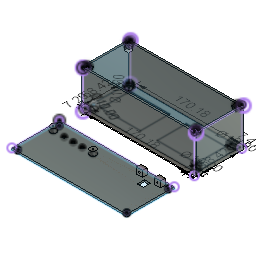
Digital Clock Enclosure v22 (Autodesk Fusion 360 design; units mm, degrees)
Autodesk Fusion 360 part; units mm, degrees
note: some values were not read from the file. Chosen so that the rebuilt part matches the saved one: which face or edge a step refers to.
sketch "Sketch1" plane through (0, 0, 0) normal (0, 0, 1) x (1, 0, 0)
  line L0 (0, 0) -> (185, 0)
  line L1 (185, 0) -> (185, 73)
  line L2 (185, 73) -> (0, 73)
  line L3 (0, 73) -> (0, 0)
  line L4 (13, 62) -> (78.5, 62)
  line L5 (78.5, 62) -> (78.5, 14)
  line L6 (78.5, 14) -> (13, 14)
  line L7 (13, 14) -> (13, 62)
  line L8 (106.5, 62) -> (172, 62)
  line L9 (172, 62) -> (172, 14)
  line L10 (172, 14) -> (106.5, 14)
  line L11 (106.5, 14) -> (106.5, 62)
  dimension "d1" = 185
  dimension "d2" = 73
  dimension "d3" = 13
  dimension "d4" = 13
  dimension "d5" = 28
  dimension "d6" = 14
  dimension "d7" = 14
  dimension "d8" = 11
  dimension "d9" = 11
  constraint horizontal L0
  constraint vertical L1
  constraint horizontal L2
  constraint vertical L3
  constraint coincident L0.start L3.end
  constraint horizontal L4
  constraint vertical L5
  constraint horizontal L6
  constraint vertical L7
  constraint horizontal L8
  constraint vertical L9
  constraint horizontal L10
  constraint vertical L11
  constraint equal L6 L10
  measures "d1" distance of L1 L3
  measures "d2" distance of L0.end L1.end
  measures "d3" distance of L1 L9
  measures "d4" distance of L3 L7
  measures "d5" distance of L5 L11
  measures "d6" distance of L0 L10
  measures "d7" distance of L0 L6
  measures "d8" distance of L2 L8
  measures "d9" distance of L2 L4
extrude "Extrude1" add sketch "Sketch1" along normal blind 60 makes body 1
shell "Shell2" thickness 3 outward yes removed faces 1 at (97.1667, 30, 60) on bodies 1
extrude "Extrude6" cut 1 faces at (129.3333, 61, 60) along direction (0, 0, -1) blind 63 on bodies 1 bodies 1
extrude "Extrude7" cut 1 faces at (55.6667, 15, 60) along direction (0, 0, -1) blind 63 on bodies 1 bodies 1
sketch "Sketch5" plane through (0, 0, 0) normal (0, 0, 1) x (-1, 0, 0)
  line L0 (-78.5, -14) -> (-13, -14)
  line L1 (-13, -14) -> (-13, -62)
  line L2 (-13, -62) -> (-78.5, -62)
  line L3 (-78.5, -62) -> (-78.5, -14)
  line L4 (-172, -14) -> (-106.5, -14)
  line L5 (-106.5, -14) -> (-106.5, -62)
  line L6 (-106.5, -62) -> (-172, -62)
  line L7 (-172, -62) -> (-172, -14)
  line L8 (0, -73) -> (0, 0)
  line L9 (0, 0) -> (-185, 0)
  line L10 (-185, 0) -> (-185, -73)
  line L11 (-185, -73) -> (0, -73)
  circle A0 centre (-7.41, -65.71) radius 5
  circle A1 centre (-7.41, -7.29) radius 5
  circle A2 centre (-177.59, -65.71) radius 5
  circle A3 centre (-177.59, -7.29) radius 5
  dimension "d26" = 10
  dimension "d27" = 10
  dimension "d28" = 10
  dimension "d29" = 10
  dimension "d30" = 170.18
  dimension "d31" = 170.18
  dimension "d32" = 58.42
  dimension "d33" = 58.42
  dimension "d34" = 7.41
  dimension "d35" = 7.41
  dimension "d36" = 7.29
  dimension "d37" = 7.29
  measures "d26" diameter of A0
  measures "d27" diameter of A1
  measures "d28" diameter of A2
  measures "d29" diameter of A3
  measures "d30" horizontal distance of A0.centre A2.centre
  measures "d31" horizontal distance of A1.centre A3.centre
  measures "d32" vertical distance of A2.centre A3.centre
  measures "d33" vertical distance of A0.centre A1.centre
  measures "d34" distance of L10 A2.centre
  measures "d35" distance of L10 A3.centre
  measures "d36" distance of L9 A3.centre
  measures "d37" distance of L9 A1.centre
extrude "Extrude8" add sketch "Sketch5" along normal blind 5 contours A0 | A1 | A2 | A3 bodies 1
sketch "Sketch10" plane through (0, 0, 0) normal (0, 0, 1) x (-1, 0, 0)
  circle A0 centre (-7.41, -65.71) radius 5
  circle A1 centre (-7.41, -7.29) radius 5
  circle A2 centre (-177.59, -65.71) radius 5
  circle A3 centre (-177.59, -7.29) radius 5
  line L0 (-78.5, -14) -> (-13, -14)
  line L1 (-13, -14) -> (-13, -62)
  line L2 (-13, -62) -> (-78.5, -62)
  line L3 (-78.5, -62) -> (-78.5, -14)
  line L4 (-172, -14) -> (-106.5, -14)
  line L5 (-106.5, -14) -> (-106.5, -62)
  line L6 (-106.5, -62) -> (-172, -62)
  line L7 (-172, -62) -> (-172, -14)
  line L8 (0, -73) -> (0, 0)
  line L9 (0, 0) -> (-185, 0)
  line L10 (-185, 0) -> (-185, -73)
  line L11 (-185, -73) -> (0, -73)
extrude "Extrude9" cut 1 faces at (5.9084, 66.4331, 5) along direction (0, 0, -1) blind 5 on bodies 1 bodies 1
sketch "Sketch11" plane through (0, 0, 0) normal (0, 0, 1) x (-1, 0, 0)
extrude "Extrude10" cut 3 faces at (176.2129, 65.2679, 5) (178.4699, 5.0481, 5) (8.3568, 6.5995, 5) along direction (0, 0, -1) blind 5 on bodies 1 bodies 1
sketch "Sketch12" plane through (0, 0, 0) normal (0, 0, 1) x (1, 0, 0)
extrude "Extrude11" add sketch "Sketch10" along normal blind 5 contours A0 | A1 | A2 | A3 bodies 1
sketch "Sketch13" plane through (0, 0, 0) normal (0, 0, 1) x (-1, 0, 0)
sketch "Sketch14" plane through (0, 0, 0) normal (0, 0, 1) x (-1, 0, 0)
sketch "Sketch15" plane through (0, 0, 0) normal (0, 0, 1) x (-1, 0, 0)
sketch "Sketch16" plane through (0, 0, 0) normal (1, 0, 0) x (0, 1, 0)
  line L0 (0, 0) -> (73, 0)
  line L1 (73, 0) -> (73, 60)
  line L2 (73, 60) -> (0, 60)
  line L3 (0, 60) -> (0, 0)
sketch "Sketch18" plane through (-3, 0, 0) normal (-1, 0, 0) x (0, -1, 0)
  line L0 (-76, -3) -> (3, -3)
  line L1 (3, -3) -> (3, 60)
  line L2 (3, 60) -> (-76, 60)
  line L3 (-76, 60) -> (-76, -3)
sketch "Sketch19" plane through (-3, 0, 0) normal (-1, 0, 0) x (0, -1, 0)
  line L0 (-76, -3) -> (3, -3)
  line L1 (3, -3) -> (3, 60)
  line L2 (3, 60) -> (-76, 60)
  line L3 (-76, 60) -> (-76, -3)
sketch "Sketch20" plane through (0, 0, 0) normal (1, 0, 0) x (0, 1, 0)
  line L0 (0, 0) -> (73, 0)
  line L1 (73, 0) -> (73, 60)
  line L2 (73, 60) -> (0, 60)
  line L3 (0, 60) -> (0, 0)
sketch "Sketch24" plane through (188, 0, 0) normal (1, 0, 0) x (0, 1, 0)
  line L0 (-3, -3) -> (76, -3)
  line L1 (76, -3) -> (76, 60)
  line L2 (76, 60) -> (-3, 60)
  line L3 (-3, 60) -> (-3, -3)
sketch "Sketch25" plane through (188, 0, 0) normal (1, 0, 0) x (0, 1, 0)
sketch "Sketch34" plane through (0, 0, 0) normal (1, 0, 0) x (0, 1, 0)
  line L0 (0, 60) -> (7, 60)
  line L1 (7, 60) -> (7, 55)
  line L2 (7, 55) -> (0, 55)
  line L3 (0, 55) -> (0, 60)
  line L4 (-3, 60) -> (-3, -3)
  point P0 (-3, 60)
  dimension "d68" = 7
  dimension "d69" = 5
  dimension "d70" = 3
  constraint horizontal L0
  constraint vertical L1
  constraint horizontal L2
  constraint vertical L3
  constraint coincident L0 P0
  measures "d68" distance of L0.start L0.end
  measures "d69" distance of L0.start L2.end
  measures "d70" distance of L3 L4
extrude "Extrude15" add sketch "Sketch34" along normal blind 7 bodies 1
move_face "MoveFace7" to x (0.642788, 0, 0.766044) y (-0.439385, 0.819152, 0.368688) z (-0.627507, -0.573576, 0.526541) at (40.0891, 32.8126, 18.0971) 1 faces at (2.3333, 4.6667, 55) on bodies 1
move_face "MoveFace8" by (-1.255, -1.1472, 1.0531) 1 faces at (2.3333, 2.3333, 44.3549) on bodies 1
sketch "Sketch35" plane through (0, 0, 0) normal (1, 0, 0) x (0, 1, 0)
  line L0 (66, 60) -> (73, 60)
  line L1 (73, 60) -> (73, 55)
  line L2 (73, 55) -> (66, 55)
  line L3 (66, 55) -> (66, 60)
  line L4 (76, -3) -> (76, 60)
  point P0 (76, 60)
  dimension "d73" = 7
  dimension "d74" = 5
  dimension "d75" = 3
  constraint horizontal L0
  constraint vertical L1
  constraint horizontal L2
  constraint vertical L3
  constraint coincident L0 P0
  measures "d73" distance of L0.start L0.end
  measures "d74" distance of L0.start L2.end
  measures "d75" distance of L1 L4
extrude "Extrude16" add sketch "Sketch35" along normal blind 7 bodies 1
move_face "MoveFace9" to x (0.642788, 0, 0.766044) y (0.439385, 0.819152, -0.368688) z (-0.627507, 0.573576, 0.526541) at (6.7589, -18.4636, 46.0644) 1 faces at (2.3333, 70.6667, 55) on bodies 1
sketch "Sketch36" plane through (185, 0, 0) normal (-1, 0, 0) x (0, -1, 0)
  line L0 (-73, 0) -> (0, 0)
  line L1 (0, 0) -> (0, 60)
  line L2 (0, 60) -> (-73, 60)
  line L3 (-73, 60) -> (-73, 0)
sketch "Sketch37" plane through (185, 0, 0) normal (-1, 0, 0) x (0, -1, 0)
  line L0 (-73, 60) -> (-66, 60)
  line L1 (-66, 60) -> (-66, 55)
  line L2 (-66, 55) -> (-73, 55)
  line L3 (-73, 55) -> (-73, 60)
  line L4 (-76, 60) -> (-76, -3)
  line L5 (-7, 60) -> (0, 60)
  line L6 (0, 60) -> (0, 55)
  line L7 (0, 55) -> (-7, 55)
  line L8 (-7, 55) -> (-7, 60)
  line L9 (3, -3) -> (3, 60)
  point P0 (-76, 60)
  point P1 (3, 60)
  dimension "d78" = 7
  dimension "d79" = 5
  dimension "d80" = 3
  dimension "d81" = 7
  dimension "d82" = 5
  dimension "d83" = 3
  constraint horizontal L0
  constraint vertical L1
  constraint horizontal L2
  constraint vertical L3
  constraint coincident L0 P0
  constraint horizontal L5
  constraint vertical L6
  constraint horizontal L7
  constraint vertical L8
  constraint coincident L5 P1
  measures "d78" distance of L0.start L0.end
  measures "d79" distance of L0.start L2.end
  measures "d80" distance of L3 L4
  measures "d81" distance of L5.start L5.end
  measures "d82" distance of L5.start L7.end
  measures "d83" distance of L6 L9
extrude "Extrude17" add sketch "Sketch37" along normal blind 7 bodies 1
move_face "MoveFace10" to x (0.642788, 0, -0.766044) y (0.439385, 0.819152, 0.368688) z (0.627507, -0.573576, 0.526541) at (27.2502, 31.6655, 160.8684) 1 faces at (182.6667, 2.3333, 55) on bodies 1
move_face "MoveFace11" to x (0.819152, -0.439385, -0.368688) y (0, 0.642788, -0.766044) z (0.573576, 0.627507, 0.526541) at (1.7914, 68.5287, 143.2787) 1 faces at (182.6667, 68.3333, 55) on bodies 1
sketch "Sketch39" plane through (0, 0, 0) normal (0, 0, 1) x (1, 0, 0)
  line L0 (-0.7205, -41.6473) -> (190.2795, -41.6473)
  line L1 (190.2795, -41.6473) -> (190.2795, -120.6473)
  line L2 (190.2795, -120.6473) -> (-0.7205, -120.6473)
  line L3 (-0.7205, -120.6473) -> (-0.7205, -41.6473)
  dimension "d86" = 191
  dimension "d87" = 79
  constraint horizontal L0
  constraint vertical L1
  constraint horizontal L2
  constraint vertical L3
  measures "d86" distance of L0.start L0.end
  measures "d87" distance of L0.start L2.end
extrude "Extrude18" add sketch "Sketch39" along normal blind 3 separate body makes body 2
sketch "Sketch41" plane through (0, 0, 0) normal (0, 0, -1) x (1, 0, 0)
  line L0 (190.2795, 120.6473) -> (-0.7205, 120.6473)
  line L1 (-0.7205, 120.6473) -> (-0.7205, 41.6473)
  line L2 (-0.7205, 41.6473) -> (190.2795, 41.6473)
  line L3 (190.2795, 41.6473) -> (190.2795, 120.6473)
  circle A0 centre (4.2795, 115.6473) radius 1.6
  circle A1 centre (4.2795, 46.6473) radius 1.6
  circle A2 centre (185.2795, 115.6473) radius 1.6
  circle A3 centre (185.2795, 46.6473) radius 1.6
  dimension "d92" = 3.2
  dimension "d93" = 3.2
  dimension "d94" = 3.2
  dimension "d95" = 3.2
  dimension "d96" = 5
  dimension "d97" = 5
  dimension "d98" = 5
  dimension "d99" = 5
  dimension "d100" = 5
  dimension "d101" = 5
  dimension "d102" = 5
  dimension "d103" = 5
  measures "d92" diameter of A0
  measures "d93" diameter of A1
  measures "d94" diameter of A2
  measures "d95" diameter of A3
  measures "d96" distance of L1 A0.centre
  measures "d97" distance of L0 A0.centre
  measures "d98" distance of L1 A1.centre
  measures "d99" distance of L2 A1.centre
  measures "d100" distance of L3 A3.centre
  measures "d101" distance of L2 A3.centre
  measures "d102" distance of L0 A2.centre
  measures "d103" distance of L3 A2.centre
extrude "Extrude19" cut sketch "Sketch41" against normal blind 3 contours A0 bodies 2
extrude "Extrude20" cut sketch "Sketch41" against normal blind 3 contours A1 bodies 2
extrude "Extrude21" cut sketch "Sketch41" against normal blind 3 contours A3 bodies 2
extrude "Extrude22" cut sketch "Sketch41" against normal blind 3 contours A2 bodies 2
sketch "Sketch42" plane through (0, 0, 0) normal (0, 0, -1) x (1, 0, 0)
  circle A0 centre (4.2795, 46.6473) radius 2.75
  circle A1 centre (4.2795, 115.6473) radius 2.75
  circle A2 centre (185.2795, 115.6473) radius 2.75
  circle A3 centre (185.2795, 46.6473) radius 2.75
  point P0 (4.2795, 46.6473)
  point P1 (4.2795, 115.6473)
  point P2 (185.2795, 115.6473)
  point P3 (185.2795, 46.6473)
  dimension "d112" = 5.5
  dimension "d113" = 5.5
  dimension "d114" = 5.5
  dimension "d115" = 5.5
  constraint coincident P0 A0.centre
  constraint coincident P1 A1.centre
  constraint coincident P2 A2.centre
  constraint coincident P3 A3.centre
  measures "d112" diameter of A0
  measures "d113" diameter of A1
  measures "d114" diameter of A2
  measures "d115" diameter of A3
extrude "Extrude23" cut sketch "Sketch42" against normal blind 2 contours A1 bodies 2
extrude "Extrude24" cut sketch "Sketch42" against normal blind 2 contours A0 bodies 2
extrude "Extrude25" cut sketch "Sketch42" against normal blind 2 contours A2 bodies 2
extrude "Extrude26" cut sketch "Sketch42" against normal blind 2 contours A3 bodies 2
sketch "Sketch43" plane through (0, 0, 3) normal (0, 0, 1) x (-1, 0, 0)
  circle A0 centre (-185.2795, 115.6473) radius 1.6
  circle A1 centre (-185.2795, 46.6473) radius 1.6
  circle A2 centre (-4.2795, 46.6473) radius 1.6
  circle A3 centre (-4.2795, 115.6473) radius 1.6
  line L0 (0.7205, 120.6473) -> (-190.2795, 120.6473)
  line L1 (-190.2795, 120.6473) -> (-190.2795, 41.6473)
  line L2 (-190.2795, 41.6473) -> (0.7205, 41.6473)
  line L3 (0.7205, 41.6473) -> (0.7205, 120.6473)
  circle A4 centre (-27.2795, 61.6473) radius 1.75
  circle A5 centre (-42.2795, 61.6473) radius 1.75
  circle A6 centre (-57.2795, 61.6473) radius 1.75
  circle A7 centre (-9.2795, 61.6473) radius 5
  circle A8 centre (-75.2795, 61.6473) radius 5
  line L4 (0.7205, 41.6473) -> (-190.2795, 41.6473)
  line L5 (0.7205, 120.6473) -> (0.7205, 41.6473)
  dimension "d124" = 3.5
  dimension "d125" = 3.5
  dimension "d126" = 3.5
  dimension "d127" = 15
  dimension "d128" = 15
  dimension "d129" = 10
  dimension "d130" = 10
  dimension "d131" = 18
  dimension "d132" = 18
  dimension "d157" = 20
  dimension "d159" = 10
  constraint horizontal A4.centre A5.centre
  constraint horizontal A5.centre A6.centre
  constraint horizontal A4.centre A7.centre
  constraint horizontal A6.centre A8.centre
  measures "d124" diameter of A4
  measures "d125" diameter of A5
  measures "d126" diameter of A6
  measures "d127" distance of A4.centre A5.centre
  measures "d128" distance of A5.centre A6.centre
  measures "d129" diameter of A7
  measures "d130" diameter of A8
  measures "d131" distance of A4.centre A7.centre
  measures "d132" distance of A6.centre A8.centre
  measures "d157" distance of A7.centre L4
  measures "d159" distance of A7.centre L5
sketch "Sketch45" plane through (0, 0, 5) normal (0, 0, 1) x (-1, 0, 0)
  circle A0 centre (-7.41, -65.71) radius 5
  circle A1 centre (-7.41, -65.71) radius 1.05
  dimension "d135" = 2.1
  constraint coincident A0.centre A1.centre
  measures "d135" diameter of A1
sketch "Sketch47" plane through (0, 0, 5) normal (0, 0, 1) x (-1, 0, 0)
  circle A0 centre (-7.41, -7.29) radius 5
  circle A1 centre (-7.4207, -7.29) radius 1.05
  dimension "d136" = 2.1
  measures "d136" diameter of A1
sketch "Sketch48" plane through (0, 0, 5) normal (0, 0, 1) x (-1, 0, 0)
  circle A0 centre (-177.59, -65.71) radius 5
  circle A1 centre (-177.59, -65.71) radius 1.05
  dimension "d137" = 2.1
  constraint coincident A0.centre A1.centre
  measures "d137" diameter of A1
sketch "Sketch49" plane through (0, 0, 5) normal (0, 0, 1) x (-1, 0, 0)
  circle A0 centre (-177.59, -7.29) radius 5
  circle A1 centre (-177.59, -7.29) radius 1.05
  dimension "d138" = 2.1
  constraint coincident A0.centre A1.centre
  measures "d138" diameter of A1
extrude "Extrude27" cut sketch "Sketch48" sketch "Sketch45" sketch "Sketch49" sketch "Sketch47" against normal blind 6 contours A1 of sketch 2 contours A1 of sketch 3 contours A1 of sketch 4 contours A1 bodies 1
sketch "Sketch50" plane through (0, 0, 60) normal (0, 0, 1) x (-1, 0, 0)
  line L0 (-7, -73) -> (-178, -73)
  line L1 (-178, -73) -> (-178, -66)
  line L2 (-178, -66) -> (-185, -66)
  line L3 (-185, -66) -> (-185, -7)
  line L4 (-185, -7) -> (-178, -7)
  line L5 (-178, -7) -> (-178, 0)
  line L6 (-178, 0) -> (-7, 0)
  line L7 (-7, 0) -> (-7, -7)
  line L8 (-7, -7) -> (0, -7)
  line L9 (0, -7) -> (0, -66)
  line L10 (0, -66) -> (-7, -66)
  line L11 (-7, -66) -> (-7, -73)
  line L12 (3, -76) -> (3, 3)
  line L13 (3, 3) -> (-188, 3)
  line L14 (-188, 3) -> (-188, -76)
  line L15 (-188, -76) -> (3, -76)
  circle A0 centre (-2, -2) radius 1.05
  circle A1 centre (-2, -71) radius 1.05
  circle A2 centre (-183, -71) radius 1.05
  line L16 (-188, -76) -> (-188, 3)
  circle A3 centre (-183, -2) radius 1.05
  dimension "d141" = 2.1
  dimension "d142" = 5
  dimension "d143" = 5
  dimension "d144" = 2.1
  dimension "d145" = 5
  dimension "d146" = 5
  dimension "d147" = 2.1
  dimension "d148" = 5
  dimension "d149" = 5
  dimension "d150" = 2.1
  dimension "d151" = 5
  dimension "d152" = 5
  measures "d141" diameter of A0
  measures "d142" distance of L12 A0.centre
  measures "d143" distance of L13 A0.centre
  measures "d144" diameter of A1
  measures "d145" distance of L12 A1.centre
  measures "d146" distance of L15 A1.centre
  measures "d147" diameter of A2
  measures "d148" distance of L15 A2.centre
  measures "d149" distance of A2.centre L16
  measures "d150" diameter of A3
  measures "d151" distance of L16 A3.centre
  measures "d152" distance of L13 A3.centre
extrude "Extrude29" cut sketch "Sketch50" against normal blind 9 contours A0 | A1 | A2 | A3 bodies 1
sketch "Sketch56" plane through (0, 0, 3) normal (0, 0, 1) x (-1, 0, 0)
sketch "Sketch57" plane through (0, 0, 3) normal (0, 0, 1) x (1, 0, 0)
sketch "Sketch58" plane through (0, 0, 3) normal (0, 0, 1) x (-1, 0, 0)
sketch "Sketch59" plane through (0, 0, 3) normal (0, 0, 1) x (1, 0, 0)
extrude "Extrude30" cut sketch "Sketch43" against normal blind 3 contours A4 | A5 | A6 bodies 2
extrude "Extrude31" add sketch "Sketch43" along normal blind 7 contours A7 | A8 bodies 2
sketch "Sketch60" plane through (0, 0, 10) normal (0, 0, 1) x (-1, 0, 0)
  circle A0 centre (-9.2795, 61.6473) radius 5
  circle A1 centre (-9.2795, 61.6473) radius 1.05
  point P0 (-9.2795, 61.6473)
  dimension "d164" = 2.1
  constraint coincident P0 A0.centre
  measures "d164" diameter of A1
extrude "Extrude32" cut sketch "Sketch60" against normal blind 7 contours A1 bodies 2
sketch "Sketch61" plane through (0, 0, 10) normal (0, 0, 1) x (-1, 0, 0)
  circle A0 centre (-75.2795, 61.6473) radius 5
  circle A1 centre (-75.2795, 61.6473) radius 1.05
  point P0 (-75.2795, 61.6473)
  dimension "d167" = 2.1
  constraint coincident P0 A0.centre
  measures "d167" diameter of A1
extrude "Extrude33" cut sketch "Sketch61" against normal blind 7 contours A1 bodies 2
sketch "Sketch62" plane through (0, 0, 3) normal (0, 0, 1) x (1, 0, 0)
  line L0 (140.2795, -46.6473) -> (150.2795, -46.6473)
  line L1 (150.2795, -46.6473) -> (150.2795, -54.6473)
  line L2 (150.2795, -54.6473) -> (140.2795, -54.6473)
  line L3 (140.2795, -54.6473) -> (140.2795, -46.6473)
  line L4 (170.2795, -46.6473) -> (180.2795, -46.6473)
  line L5 (180.2795, -46.6473) -> (180.2795, -54.6473)
  line L6 (180.2795, -54.6473) -> (170.2795, -54.6473)
  line L7 (170.2795, -54.6473) -> (170.2795, -46.6473)
  line L8 (-0.7205, -41.6473) -> (190.2795, -41.6473)
  line L9 (190.2795, -41.6473) -> (190.2795, -120.6473)
  dimension "d170" = 10
  dimension "d171" = 8
  dimension "d172" = 10
  dimension "d173" = 8
  dimension "d174" = 5
  dimension "d175" = 20
  dimension "d176" = 10
  constraint horizontal L0
  constraint vertical L1
  constraint horizontal L2
  constraint vertical L3
  constraint horizontal L4
  constraint vertical L5
  constraint horizontal L6
  constraint vertical L7
  constraint horizontal L0.end L4.start
  measures "d170" distance of L0.start L0.end
  measures "d171" distance of L0.start L2.end
  measures "d172" distance of L4.start L4.end
  measures "d173" distance of L4.start L6.end
  measures "d174" distance of L4 L8
  measures "d175" distance of L1 L7
  measures "d176" distance of L5 L9
extrude "Extrude34" add sketch "Sketch62" along normal blind 10 bodies 2
sketch "Sketch63" plane through (0, -54.6473, 0) normal (0, -1, 0) x (1, 0, 0)
  line L0 (140.2795, 3) -> (150.2795, 3)
  line L1 (150.2795, 3) -> (150.2795, 13)
  line L2 (150.2795, 13) -> (140.2795, 13)
  line L3 (140.2795, 13) -> (140.2795, 3)
  circle A0 centre (145.2795, 8) radius 1.05
  dimension "d179" = 2.1
  dimension "d180" = 5
  dimension "d181" = 5
  measures "d179" diameter of A0
  measures "d180" distance of L2 A0.centre
  measures "d181" distance of L3 A0.centre
sketch "Sketch64" plane through (0, -54.6473, 0) normal (0, -1, 0) x (1, 0, 0)
  line L0 (170.2795, 3) -> (180.2795, 3)
  line L1 (180.2795, 3) -> (180.2795, 13)
  line L2 (180.2795, 13) -> (170.2795, 13)
  line L3 (170.2795, 13) -> (170.2795, 3)
  circle A0 centre (175.2795, 8) radius 1.05
  dimension "d182" = 2.1
  dimension "d183" = 5
  dimension "d184" = 5
  measures "d182" diameter of A0
  measures "d183" distance of L3 A0.centre
  measures "d184" distance of L2 A0.centre
extrude "Extrude35" cut sketch "Sketch64" sketch "Sketch63" against normal blind 6 contours A0 of sketch 2 contours A0 bodies 2
sketch "Sketch65" plane through (0, 0, 3) normal (0, 0, 1) x (1, 0, 0)
  line L0 (155.2795, -56.2473) -> (165.2795, -56.2473)
  line L1 (165.2795, -56.2473) -> (165.2795, -68.2473)
  line L2 (165.2795, -68.2473) -> (155.2795, -68.2473)
  line L3 (155.2795, -68.2473) -> (155.2795, -56.2473)
  line L4 (150.2795, -46.6473) -> (150.2795, -54.6473)
  line L5 (150.2795, -54.6473) -> (140.2795, -54.6473)
  dimension "d187" = 10
  dimension "d188" = 12
  dimension "d189" = 5
  dimension "d190" = 1.6
  constraint horizontal L0
  constraint vertical L1
  constraint horizontal L2
  constraint vertical L3
  measures "d187" distance of L0.start L0.end
  measures "d188" distance of L0.start L2.end
  measures "d189" distance of L3 L4
  measures "d190" distance of L0 L5
extrude "Extrude36" cut sketch "Sketch65" against normal blind 3 bodies 2
sketch "Sketch51" plane through (0, 0, 60) normal (0, 0, 1) x (1, 0, 0)
sketch "Sketch52" plane through (0, 0, 0) normal (0, 0, 1) x (1, 0, 0)
sketch "Sketch53" plane through (0, 0, 3) normal (0, 0, 1) x (-1, 0, 0)
sketch "Sketch54" plane through (0, 0, 3) normal (0, 0, 1) x (1, 0, 0)
sketch "Sketch55" plane through (0, 0, 3) normal (0, 0, 1) x (1, 0, 0)
extrude "Extrude28" [suppressed]
sketch "Sketch40" plane through (0, 0, 3) normal (0, 0, 1) x (-1, 0, 0)
  line L0 (0.7205, 120.6473) -> (-190.2795, 120.6473)
  line L1 (-190.2795, 120.6473) -> (-190.2795, 41.6473)
  line L2 (-190.2795, 41.6473) -> (0.7205, 41.6473)
  line L3 (0.7205, 41.6473) -> (0.7205, 120.6473)
  circle A0 centre (-3.1706, 115.8043) radius 1.6
  circle A1 centre (-5.0524, 47.4308) radius 1.6
  dimension "d90" = 3.2
  dimension "d91" = 3.2
  measures "d90" diameter of A0
  measures "d91" diameter of A1
sketch "Sketch38" plane through (0, 0, 55) normal (0, 0, -1) x (1, 0, 0)
  line L0 (185, -73) -> (185, -66)
  line L1 (185, -66) -> (178, -66)
  line L2 (178, -66) -> (178, -73)
  line L3 (178, -73) -> (185, -73)
sketch "Sketch32" plane through (0, 0, 0) normal (1, 0, 0) x (0, 1, 0)
  line L0 (-1.7668, 60) -> (5.2332, 60)
  line L1 (5.2332, 60) -> (5.2332, 55)
  line L2 (5.2332, 55) -> (-1.7668, 55)
  line L3 (-1.7668, 55) -> (-1.7668, 60)
  point P0 (-3, 60)
  dimension "d65" = 7
  dimension "d66" = 5
  constraint horizontal L0
  constraint vertical L1
  constraint horizontal L2
  constraint vertical L3
  constraint coincident L0 P0
  measures "d65" distance of L0.start L0.end
  measures "d66" distance of L0.start L2.end
sketch "Sketch33" plane through (0, 0, 0) normal (1, 0, 0) x (0, 1, 0)
  line L0 (-1.7668, 55) -> (-1.7668, 60)
  line L1 (-3, 60) -> (-3, -3)
sketch "Sketch26" plane through (0, 0, 0) normal (1, 0, 0) x (0, 1, 0)
  line L0 (0, 60) -> (10, 60)
  line L1 (10, 60) -> (10, 55)
  line L2 (10, 55) -> (0, 55)
  line L3 (0, 55) -> (0, 60)
  line L4 (-3, 60) -> (-3, -3)
  point P0 (-3, 60)
  dimension "d54" = 10
  dimension "d55" = 5
  dimension "d56" = 3
  constraint horizontal L0
  constraint vertical L1
  constraint horizontal L2
  constraint vertical L3
  constraint coincident L0 P0
  measures "d54" distance of L0.start L0.end
  measures "d55" distance of L0.start L2.end
  measures "d56" distance of L3 L4
sketch "Sketch31" plane through (0, 0, 0) normal (1, 0, 0) x (0, 1, 0)
extrude "Extrude12" [suppressed]
sketch "Sketch30" plane through (10, 0, 0) normal (1, 0, 0) x (0, 1, 0)
  line L0 (0, 55) -> (10, 55)
  line L1 (10, 55) -> (10, 60)
  line L2 (10, 60) -> (0, 60)
  line L3 (0, 60) -> (0, 55)
fillet "Fillet1" [suppressed]
other "Form2"
other "Form3"
sketch "Sketch29" plane through (0, 0, 0) normal (0, 0, 1) x (1, 0, 0)
extrude "Extrude13" [suppressed]
extrude "Extrude14" [suppressed]
moveface "MoveFace6" [suppressed]
moveface "MoveFace5" [suppressed]
moveface "MoveFace2" [suppressed]
moveface "MoveFace3" [suppressed]
moveface "MoveFace4" [suppressed]
moveface "MoveFace1" [suppressed]
sketch "Sketch27" plane through (0, 0, 55) normal (0, 0, -1) x (1, 0, 0)
  arc A0 (4, -10) -> (10, -4) centre (4, -4) ccw
  line L0 (10, -4) -> (10, 0)
  line L1 (10, 0) -> (0, 0)
  line L2 (0, 0) -> (0, -10)
  line L3 (0, -10) -> (4, -10)
  arc A1 (4, -10) -> (10, -4) centre (4, -4) ccw
  line L4 (10, -4) -> (10, 0)
  line L5 (0, 0) -> (10, 0)
  line L6 (0, -10) -> (0, 0)
  line L7 (0, -73) -> (0, -10)
  line L8 (185, -73) -> (0, -73)
  line L9 (185, 0) -> (185, -73)
  line L10 (10, 0) -> (185, 0)
  line L11 (0, -10) -> (4, -10)
  line L12 (-3, -76) -> (188, -76)
  line L13 (188, -76) -> (188, 3)
  line L14 (188, 3) -> (-3, 3)
  line L15 (-3, 3) -> (-3, -76)
sketch "Sketch28" plane through (0, 0, 55) normal (0, 0, -1) x (1, 0, 0)
  arc A0 (4, -10) -> (10, -4) centre (4, -4) ccw
  line L0 (10, -4) -> (10, 0)
  line L1 (0, 0) -> (10, 0)
  line L2 (0, -10) -> (0, 0)
  line L3 (0, -73) -> (0, -10)
  line L4 (185, -73) -> (0, -73)
  line L5 (185, 0) -> (185, -73)
  line L6 (10, 0) -> (185, 0)
  line L7 (0, -10) -> (4, -10)
  line L8 (-3, -76) -> (188, -76)
  line L9 (188, -76) -> (188, 3)
  line L10 (188, 3) -> (-3, 3)
  line L11 (-3, 3) -> (-3, -76)
sketch "Sketch6" plane through (0, 0, 5) normal (0, 0, 1) x (-1, 0, 0)
  circle A0 centre (-7.41, -65.71) radius 3.5
sketch "Sketch7" plane through (0, 0, 5) normal (0, 0, 1) x (-1, 0, 0)
other "Form1"
sketch "Sketch8" plane through (0, 0, 5) normal (0, 0, 1) x (-1, 0, 0)
hole "Hole1" [suppressed]
sketch "Sketch9" plane through (0, 0, 5) normal (0, 0, 1) x (-1, 0, 0)
  circle A0 centre (-7.41, -7.29) radius 3.5
extrude "Extrude4" [suppressed]
extrude "Extrude5" [suppressed]
sketch "Sketch4" plane through (0, 0, 0) normal (0, 0, 1) x (-1, 0, 0)
  line L0 (-169, -17) -> (-109.5, -17)
  line L1 (-109.5, -17) -> (-109.5, -59)
  line L2 (-109.5, -59) -> (-169, -59)
  line L3 (-169, -59) -> (-169, -17)
  line L4 (-75.5, -17) -> (-16, -17)
  line L5 (-16, -17) -> (-16, -59)
  line L6 (-16, -59) -> (-75.5, -59)
  line L7 (-75.5, -59) -> (-75.5, -17)
  line L8 (0, -73) -> (0, 0)
  line L9 (0, 0) -> (-185, 0)
  line L10 (-185, 0) -> (-185, -73)
  line L11 (-185, -73) -> (0, -73)
sketch "Sketch3" plane through (0, 0, 0) normal (0, 0, 1) x (-1, 0, 0)
  line L0 (-169, -17) -> (-109.5, -17)
  line L1 (-109.5, -17) -> (-109.5, -59)
  line L2 (-109.5, -59) -> (-169, -59)
  line L3 (-169, -59) -> (-169, -17)
  line L4 (-75.5, -17) -> (-16, -17)
  line L5 (-16, -17) -> (-16, -59)
  line L6 (-16, -59) -> (-75.5, -59)
  line L7 (-75.5, -59) -> (-75.5, -17)
  line L8 (0, -73) -> (0, 0)
  line L9 (0, 0) -> (-185, 0)
  line L10 (-185, 0) -> (-185, -73)
  line L11 (-185, -73) -> (0, -73)
shell "Shell1" [suppressed]
extrude "Extrude2" [suppressed]
extrude "Extrude3" [suppressed]
sketch "Sketch2" plane through (0, 0, 3) normal (0, 0, 1) x (-1, 0, 0)
  line L0 (-81.5, -11) -> (-10, -11)
  line L1 (-10, -11) -> (-10, -65)
  line L2 (-10, -65) -> (-81.5, -65)
  line L3 (-81.5, -65) -> (-81.5, -11)
  line L4 (-175, -11) -> (-103.5, -11)
  line L5 (-103.5, -11) -> (-103.5, -65)
  line L6 (-103.5, -65) -> (-175, -65)
  line L7 (-175, -65) -> (-175, -11)
  line L8 (-3, -70) -> (-3, -3)
  line L9 (-3, -3) -> (-182, -3)
  line L10 (-182, -3) -> (-182, -70)
  line L11 (-182, -70) -> (-3, -70)
